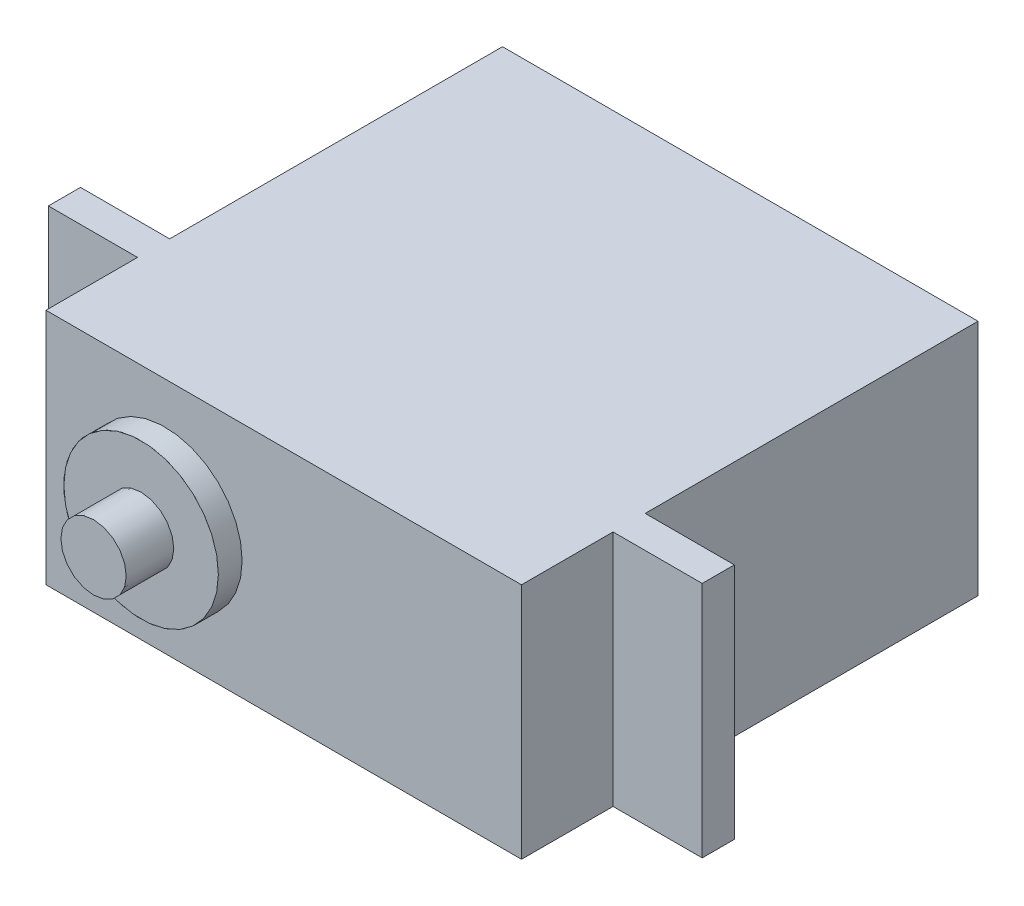
# Autodesk Inventor part: Servo2
Saved by Autodesk Inventor 2015 (Build 190159000, 159)
## iProperties
Created: 2013-12-02
Part Number: Servo2
Material: Genérico
Document SubType Name: Modeling
Designer: Gregorio
Density: 1 g/cm^3
Appearance: Valor por defecto
Author: Gregorio
Autodesk Inventor part; units mm, degrees
ref_plane "YZ Plane" through (0, 0, 0) normal (1, 0, 0) x (0, 1, 0)
ref_plane "XZ Plane" through (0, 0, 0) normal (0, 1, 0) x (-1, 0, 0)
ref_plane "XY Plane" through (0, 0, 0) normal (0, 0, 1) x (1, 0, 0)
sketch "Boceto1" plane through (0, 0, 0) normal (0, 0, 1) x (1, 0, 0)
  line L0 (0, 0) -> (40, 0)
  line L1 (40, 0) -> (40, 20)
  line L2 (40, 20) -> (0, 20)
  line L3 (0, 20) -> (0, 0)
  dimension "d0" = 40
  dimension "d1" = 20
  constraints: 8 end point, 2 parallel, 1 horizontal, 1 perpendicular
  measures "d0" distance of L2.end L1.end
  measures "d1" distance of L1.end L0.end
extrude "Extrusión1" add sketch "Boceto1" along normal blind 28
sketch "Boceto2" plane through (0, 0, 28) normal (0, 0, 1) x (1, 0, 0)
  line L0 (0, 0) -> (40, 0) projected
  line L1 (-7.5, 20) -> (47.5, 20)
  line L2 (47.5, 20) -> (47.5, 0)
  line L3 (47.5, 0) -> (-7.5, 0)
  line L4 (-7.5, 0) -> (-7.5, 20)
  point P0 (20, 0)
  point P1 (20, 0)
  dimension "d4" = 55
  constraints: 8 end point, 2 midpoint, 2 parallel, 1 coincident, 1 horizontal, 1 perpendicular
  measures "d4" distance of L2.end L3.end
extrude "Extrusión2" add sketch "Boceto2" along normal blind 2.7
sketch "Boceto3" plane through (0, 0, 30.7) normal (0, 0, 1) x (1, 0, 0)
  line L0 (0, 0) -> (40, 0)
  line L1 (40, 0) -> (40, 20)
  line L2 (40, 20) -> (0, 20)
  line L3 (0, 20) -> (0, 0)
  dimension "d7" = 40
  dimension "d8" = 20
  constraints: 8 end point, 2 parallel, 1 horizontal, 1 perpendicular
  measures "d7" distance of L2.end L1.end
  measures "d8" distance of L1.end L0.end
extrude "Extrusión3" add sketch "Boceto3" along normal blind 7.7
sketch "Boceto4" plane through (0, 0, 38.4) normal (0, 0, 1) x (1, 0, 0)
  line L0 (0, 20) -> (0, 0) projected
  circle A0 centre (10, 10) radius 6.5
  dimension "d11" = 13
  dimension "d12" = 10
  constraints: 1 centre point
  measures "d11" diameter of A0
  measures "d12" distance from line of L0 A0.centre
extrude "Extrusión4" add sketch "Boceto4" along normal blind 2
sketch "Boceto5" plane through (10, 10, 40.4) normal (0, 0, 1) x (1, 0, 0)
  circle A0 centre (0, 0) radius 6.5 projected
  circle A1 centre (0, 0) radius 2.75
  point P0 (-10, -10)
  dimension "d15" = 5.5
  constraints: 1 centre point, 1 coincident
  measures "d15" diameter of A1
extrude "Extrusión5" add sketch "Boceto5" along normal blind 4 contours A1
